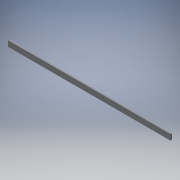
# Autodesk Inventor part: 2018 Slide
Saved by Autodesk Inventor 2018 (Build 220112000, 112)
## iProperties
Created: 2018-01-28
Part Number: 2018 Slide
Material: Generic
Document SubType Name: Modeling
Designer: Apple
Density: 1 g/cm^3
Appearance: Default
Author: Apple
Autodesk Inventor part; units mm, degrees
ref_plane "YZ Plane" through (0, 0, 0) normal (1, 0, 0) x (0, 1, 0)
ref_plane "XZ Plane" through (0, 0, 0) normal (0, 1, 0) x (-1, 0, 0)
ref_plane "XY Plane" through (0, 0, 0) normal (0, 0, 1) x (1, 0, 0)
sketch "Sketch1" plane through (0, 0, 0) normal (0, 0, 1) x (1, 0, 0)
  line L0 (-396.7005, -28.3314) -> (327.1995, -28.3314)
  line L1 (327.1995, -28.3314) -> (327.1995, -2.9314)
  line L2 (327.1995, -2.9314) -> (-396.7005, -2.9314)
  line L3 (-396.7005, -2.9314) -> (-396.7005, -28.3314)
  point P0 (0, 0)
  dimension "d0" = 723.9
  dimension "d1" = 25.4
  constraints: 8 end point, 2 perpendicular, 1 horizontal
  measures "d0" distance of L0.start L0.end
  measures "d1" distance of L0.end L1.end
extrude "Extrusion1" add sketch "Sketch1" along normal blind 6.35
body "Solid1"
